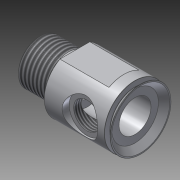
# Autodesk Inventor part: Rebuild Shooter NCDME075-0600 Cylinder Front Section
Saved by Autodesk Inventor 2014 SP1 (Build 180222100, 222)
## iProperties
Created: 2013-12-19
Part Number: Rebuild Shooter NCDME075-0600 Cylinder Front Section
Material: Aluminum 6061
Document SubType Name: Modeling
Designer: Moses
Mass: 19.3044 g
Surface Area: 41.5313 cm^2
Volume: 7.12338 cm^3
Density: 2.71 g/cm^3
Appearance: Aluminum - Flat
Author: Moses
Autodesk Inventor part; units mm, degrees
ref_plane "YZ Plane" through (0, 0, 0) normal (1, 0, 0) x (0, 1, 0)
ref_plane "XZ Plane" through (0, 0, 0) normal (0, 1, 0) x (-1, 0, 0)
sketch "Sketch1" plane through (0, 0, 0) normal (0, 0, 1) x (1, 0, 0)
  line L0 (0, 0) -> (36.195, 0)
  line L1 (0, 7.9375) -> (10.414, 7.9375)
  line L2 (10.414, 7.9375) -> (10.414, 7.9248)
  line L3 (10.414, 7.9248) -> (12.7, 7.9248)
  line L4 (12.7, 7.9248) -> (12.7, 9.525)
  line L5 (12.7, 9.525) -> (30.1625, 9.525)
  line L6 (30.1625, 9.525) -> (30.1625, 10.922)
  line L7 (30.1625, 10.922) -> (34.163, 10.922)
  line L8 (34.163, 10.922) -> (34.163, 8.89)
  line L9 (34.163, 8.89) -> (36.195, 10.922)
  line L10 (36.195, 10.922) -> (36.195, 5.715)
  line L11 (0, 7.9375) -> (0, 4.445)
  line L12 (0, 3.175) -> (12.065, 3.175)
  line L13 (36.195, 5.715) -> (36.195, 0) construction
  line L14 (0, 3.175) -> (0, 0) construction
  line L15 (34.163, 10.922) -> (36.195, 10.922) construction
  line L16 (30.1625, 8.89) -> (34.163, 8.89) construction
  line L17 (12.7, 9.525) -> (12.7, 10.922)
  line L18 (12.7, 10.922) -> (30.1625, 10.922)
  circle A0 centre (25.4, 0) radius 4.7625
  line L19 (17.145, 3.175) -> (17.145, 5.715)
  line L20 (17.145, 5.715) -> (34.163, 5.715)
  line L21 (36.195, 10.3832) -> (34.163, 8.3512)
  line L22 (34.163, 8.3512) -> (34.163, 5.715)
  line L23 (34.163, 8.89) -> (34.163, 8.3512) construction
  line L24 (34.163, 5.715) -> (36.195, 5.715) construction
  line L25 (0, 4.445) -> (12.065, 4.445)
  line L26 (12.065, 4.445) -> (12.065, 3.175)
  line L27 (12.065, 3.175) -> (17.145, 3.175)
  line L28 (0, 4.445) -> (0, 3.175)
  dimension "d0" = 17.4625
  dimension "d2" = 15.8496
  dimension "d3" = 15.875
  dimension "d4" = 2.286
  dimension "d5" = 12.7
  dimension "d6" = 6.35
  dimension "d7" = 19.05
  dimension "d8" = 21.844
  dimension "d9" = 17.78
  dimension "d10" = 45
  dimension "d11" = 36.195
  dimension "d23" = 9.525
  dimension "d24" = 25.4
  dimension "d34" = 11.43
  dimension "d35" = 19.05
  dimension "d36" = 0.381
  dimension "d45" = 12.065
  dimension "d46" = 8.89
  constraints: 58 end point, 14 vertical, 12 horizontal, 3 point on line, 1 centre point, 1 parallel
  measures "d0" distance of L4.end L5.end
  measures "d2" diameter of L2.end L0
  measures "d3" diameter of L1.start L0
  measures "d4" distance of L2.end L3.end
  measures "d5" distance of L1.start L3.end
  measures "d6" diameter of L12.start L0
  measures "d7" diameter of L5 L0
  measures "d8" diameter of L7 L0
  measures "d9" diameter of L8.end L0
  measures "d10" angle of L9 L8
  measures "d11" distance of L0.start L0.end
  measures "d23" diameter of A0
  measures "d24" distance from line of A0.centre L14
  measures "d34" diameter of L19.end L0
  measures "d35" distance of L10.end L19.end
  measures "d36" distance between parallel lines of L21 L9
  measures "d45" distance of L11.end L25.end
  measures "d46" diameter of L11.end L0
revolve "Revolution1" add sketch "Sketch1" angle 360 about axis through (0, 0, 0) along (1, 0, 0) contours L1 L2 L3 L4 L5 L6 L7 L8 L9 L10 L21 L22 L20 L19 L27 L26 L25 L11 | L17 L18 L6 L5
extrude "Extrusion1" cut sketch "Sketch1" along normal through all both and the other way through all contours L17 L18 L6 L5
extrude "Extrusion2" cut sketch "Sketch1" along normal through all contours A0 L0 | L0 A0
thread "Thread1" size "5/8-18 UNF" class "2A" standard "ANSI Unified Screw Threads" full length
chamfer "Chamfer1" distance 0.508 angle 45 2 edges at (12.7, -7.9248, 0) (0, -7.9375, 0)
chamfer "Chamfer2" distance 0.762 angle 45 1 edges at (20.6375, 0.0005, 10.922)
pattern_circular "Circular Pattern1" count 2 over 360 about axis through (21.4313, 0, 0) along (1, 0, 0) of "Extrusion1"
thread "Thread3" size "1/8" designation "1/8 - 27 NPT" standard "NPT" length 9.9568
fillet "Fillet1" radius 0.0508 6 edges at (36.195, -10.922, 0) (34.163, -8.89, 0) (34.163, -10.922, 0) (30.1625, 10.567, 2.7621) (30.1625, 10.567, -2.7621) (30.1625, -10.922, 0)
ref_plane "Work Plane1" through (21.4313, 0, 10.922) normal (0, 0, 1) x (1, 0, 0)
sketch "Sketch2" plane through (21.4313, 0, 10.922) normal (0, 0, 1) x (1, 0, 0)
  circle A0 centre (3.9687, 0.0595) radius 6.35
  line L0 (3.9687, 0.0595) -> (3.9687, -4.7625) construction
  point P0 (-21.4313, 0)
  dimension "d41" = 12.7
  dimension "d44" = 4.822
  constraints: 2 end point, 1 centre point, 1 vertical, 1 other
  measures "d41" diameter of A0
  measures "d44" distance of L0.start L0.end
extrude "Extrusion4" cut sketch "Sketch2" against normal blind 2.54
body "Solid1"
